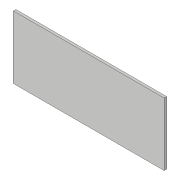
# Autodesk Inventor part: wall_plate_750 v2
Saved by Autodesk Inventor 2018 (Build 220112000, 112)
## iProperties
Created: 2017-08-23
Part Number: wall_plate_750 v2
Material: Copper
Document SubType Name: Modeling
Designer: Platform
Density: 8.94 g/cm^3
Appearance: Default
Author: Platform
Autodesk Inventor part; units mm, degrees
ref_plane "YZ Plane" through (0, 0, 0) normal (1, 0, 0) x (0, 1, 0)
ref_plane "XZ Plane" through (0, 0, 0) normal (0, 1, 0) x (-1, 0, 0)
ref_plane "XY Plane" through (0, 0, 0) normal (0, 0, 1) x (1, 0, 0)
sketch "Sketch5" plane through (0, 0, 0) normal (0, 0, 1) x (1, 0, 0)
  line L0 (0, 0) -> (0, 250)
  line L1 (0, 0) -> (250, 0) construction
  line L2 (0, 250) -> (600, 250)
  line L3 (600, 250) -> (600, 0)
  line L4 (600, 0) -> (0, 0)
  dimension "d3" = 250
  dimension "d4" = 90
  dimension "d5" = 600
  dimension "d6" = 90
  dimension "d7" = 250
  dimension "d8" = 90
  constraints: 10 end point, 3 perpendicular, 1 horizontal, 1 vertical
  measures "d3" distance of L0.start L0.end
  measures "d4" angle of L1 L0
  measures "d5" distance of L0.end L2.end
  measures "d6" angle of L0 L2
  measures "d7" distance of L2.end L3.end
  measures "d8" angle of L2 L3
extrude "Extrusion1" add sketch "Sketch5" along normal blind 10
body "Solid2"
